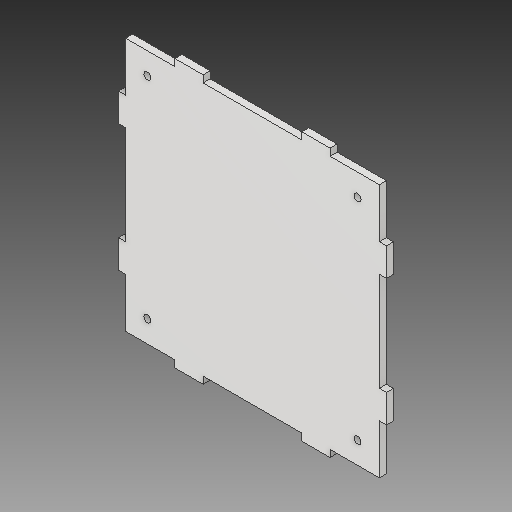
# Autodesk Inventor part: Back
Saved by Autodesk Inventor 2018.2 (Build 222227000, 227)
## iProperties
Created: 2018-04-16
Part Number: Back
Material: ABS Plastic
Document SubType Name: Modeling
Designer: Derek Fronek
Density: 1.06 g/cm^3
Appearance: Smooth - White
Author: Derek Fronek
Autodesk Inventor part; units mm, degrees
ref_plane "YZ Plane" through (0, 0, 0) normal (1, 0, 0) x (0, 1, 0)
ref_plane "XZ Plane" through (0, 0, 0) normal (0, 1, 0) x (-1, 0, 0)
ref_plane "XY Plane" through (0, 0, 0) normal (0, 0, 1) x (1, 0, 0)
sketch "Sketch1" plane through (0, 0, 0) normal (0, 0, 1) x (1, 0, 0)
  line L0 (34.925, -114.3) -> (12.7, -114.3) projected
  line L1 (34.925, -92.075) -> (34.925, -114.3) projected
  line L2 (38.1, -92.075) -> (34.925, -92.075) projected
  line L3 (38.1, -79.375) -> (38.1, -92.075) projected
  line L4 (34.925, -79.375) -> (38.1, -79.375) projected
  line L5 (34.925, -34.925) -> (34.925, -79.375) projected
  line L6 (38.1, -34.925) -> (34.925, -34.925) projected
  line L7 (38.1, -22.225) -> (38.1, -34.925) projected
  line L8 (34.925, -22.225) -> (38.1, -22.225) projected
  line L9 (34.925, 0) -> (34.925, -22.225) projected
  line L10 (12.7, 0) -> (34.925, 0) projected
  line L11 (12.7, 3.175) -> (12.7, 0) projected
  line L12 (0, 3.175) -> (12.7, 3.175) projected
  line L13 (0, 0) -> (0, 3.175) projected
  line L14 (-44.45, 0) -> (0, 0) projected
  line L15 (-44.45, 3.175) -> (-44.45, 0) projected
  line L16 (-57.15, 3.175) -> (-44.45, 3.175) projected
  line L17 (-57.15, 0) -> (-57.15, 3.175) projected
  line L18 (-79.375, 0) -> (-57.15, 0) projected
  line L19 (-79.375, -22.225) -> (-79.375, 0) projected
  line L20 (-82.55, -22.225) -> (-79.375, -22.225) projected
  line L21 (-82.55, -34.925) -> (-82.55, -22.225) projected
  line L22 (-79.375, -34.925) -> (-82.55, -34.925) projected
  line L23 (-79.375, -79.375) -> (-79.375, -34.925) projected
  line L24 (-82.55, -79.375) -> (-79.375, -79.375) projected
  line L25 (-82.55, -92.075) -> (-82.55, -79.375) projected
  line L26 (-79.375, -92.075) -> (-82.55, -92.075) projected
  line L27 (-79.375, -114.3) -> (-79.375, -92.075) projected
  line L28 (-57.15, -114.3) -> (-79.375, -114.3) projected
  line L29 (-57.15, -117.475) -> (-57.15, -114.3) projected
  line L30 (-44.45, -117.475) -> (-57.15, -117.475) projected
  line L31 (-44.45, -114.3) -> (-44.45, -117.475) projected
  line L32 (0, -114.3) -> (-44.45, -114.3) projected
  line L33 (0, -117.475) -> (0, -114.3) projected
  line L34 (12.7, -117.475) -> (0, -117.475) projected
  line L35 (12.7, -114.3) -> (12.7, -117.475) projected
  circle A0 centre (-69.5325, -9.8425) radius 1.6 projected
  circle A1 centre (25.0825, -9.8425) radius 1.6 projected
  circle A2 centre (25.0825, -104.4575) radius 1.6 projected
  circle A3 centre (-69.5325, -104.4575) radius 1.6 projected
extrude "Extrusion1" add sketch "Sketch1" along normal blind 3.175
body "Solid1"
